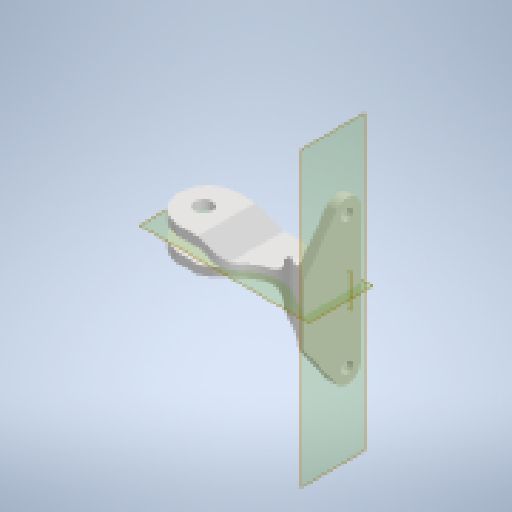
# Autodesk Inventor part: AcopleCamara-part2
Saved by Autodesk Inventor 2023 (Build 270158000, 158)
## iProperties
Created: 2023-12-18
Part Number: AcopleCamara-part2
Material: Genérico
Document SubType Name: Modeling
Designer: ASUS
Density: 1 g/cm^3
Appearance: Valor por defecto
Author: ASUS
Autodesk Inventor part; units mm, degrees
ref_plane "YZ Plane" through (0, 0, 0) normal (1, 0, 0) x (0, 1, 0)
ref_plane "XZ Plane" through (0, 0, 0) normal (0, 1, 0) x (-1, 0, 0)
ref_plane "XY Plane" through (0, 0, 0) normal (0, 0, 1) x (1, 0, 0)
ref_plane "Plano de trabajo1" through (-5.5, 31.0579, -5.3088) normal (0, 0, -1) x (0, -1, 0)
sketch "Boceto1" plane through (0, 0, -5.3088) normal (0, 0, 1) x (1, 0, 0)
  line L0 (-3, 28.0579) -> (-10.9599, 26.1093) projected
  line L1 (-3, 34.0579) -> (-3, 28.0579) projected
  line L2 (-10.9599, 36.0066) -> (-3, 34.0579) projected
  line L3 (-10.9599, 26.1093) -> (-10.9599, 36.0066) projected
  line L4 (-3, 34.0579) -> (-3, 62.1159) projected
  line L5 (-3, 0) -> (-3, 28.0579) projected
  line L6 (-11.1599, 36.2645) -> (-11.1599, 25.8544)
  line L7 (-3.2, 0) -> (-3.2, 28.009)
  line L8 (-3.2, 28.009) -> (-3.2, 28.0579)
  line L9 (-11.1599, 25.8544) -> (-3.2, 27.8031)
  line L10 (-3, 27.852) -> (-2.9524, 27.8637)
  line L11 (-3.2, 34.0579) -> (-3.2, 34.1069)
  line L12 (-3.2, 28.0579) -> (-3.2, 62.1189)
  line L13 (-2.9524, 34.2522) -> (-3, 34.2638)
  line L14 (-3.2, 34.3159) -> (-11.1599, 36.2645)
  arc A0 (-60.3157, 26.6827) -> (-60.3209, 35.4723) centre (-90.5, 31.0595) ccw projected
  arc A1 (-57.3658, 26.1226) -> (-57.3864, 36.1324) centre (-90.5, 31.0595) ccw projected
  line L15 (-60, 31.0595) -> (-57, 31.0595) construction
  line L16 (-12.8167, 21.8544) -> (-3.2, 21.8544)
  line L17 (-15.1599, 24.1976) -> (-15.1599, 37.9214)
  line L18 (-12.8167, 21.8544) -> (-15.1599, 24.1976)
  line L19 (-12.8167, 40.2645) -> (-3.2, 40.2645)
  line L20 (-12.8167, 40.2645) -> (-15.1599, 37.9214)
  line L21 (-57, 31.0595) -> (-11.1599, 31.0595) construction
  line L22 (-52.0001, 29.0595) -> (-52.0001, 33.0595)
  line L23 (-52.0001, 28.7595) -> (-37.0001, 28.7595)
  line L24 (-47.0001, 29.0595) -> (-42.0001, 29.0595)
  line L25 (-42.0001, 29.0595) -> (-42.0001, 33.0595)
  line L26 (-42.0001, 33.0595) -> (-47.0001, 33.0595)
  line L27 (-47.0001, 33.0595) -> (-47.0001, 29.0595)
  line L28 (-52.0001, 25.7595) -> (-37.0001, 25.7595)
  line L29 (-52.0001, 25.7595) -> (-52.0001, 28.7595)
  line L30 (-37.0001, 28.7595) -> (-37.0001, 33.0595) construction
  line L31 (-37.0001, 28.7595) -> (-36.5001, 28.7595)
  line L32 (-37.0001, 25.7595) -> (-27.9334, 29.0595)
  line L33 (-52.0001, 29.0595) -> (-37.0001, 29.0595)
  line L34 (-27.9334, 29.0595) -> (-15.1599, 29.0595)
  line L35 (-52.0001, 33.3595) -> (-37.0001, 33.3595)
  line L36 (-52.0001, 36.3595) -> (-37.0001, 36.3595)
  line L37 (-52.0001, 36.3595) -> (-52.0001, 33.3595)
  line L38 (-37.0001, 33.3595) -> (-36.5001, 33.3595)
  line L39 (-37.0001, 36.3595) -> (-27.9334, 33.0595)
  line L40 (-52.0001, 33.0595) -> (-37.0001, 33.0595)
  line L41 (-27.9334, 33.0595) -> (-15.1599, 33.0595)
  line L42 (-36.5001, 28.7595) -> (-30.1809, 31.0595)
  line L43 (-36.5001, 33.3595) -> (-30.1809, 31.0595)
  point P0 (0, 0)
  point P1 (-57.0001, 31.1283)
  point P2 (-47.0001, 31.0595)
  dimension "d0" = 0.2
  dimension "d3" = 4
  dimension "d7" = 4
  dimension "d9" = 4
  dimension "d10" = 5
  dimension "d12" = 5
  dimension "d13" = 5
  dimension "d14" = 15
  dimension "d15" = 3
  constraints: 76 end point, 16 parallel, 14 point on line, 10 symmetric about line, 9 horizontal, 5 vertical, 3 point on circle, 2 midpoint, 2 perpendicular, 1 other
  measures "d0" distance between parallel lines of L3 L6
  measures "d3" distance from line of L6.end L16
  measures "d7" distance between parallel lines of L6 L17
  measures "d9" distance from line of L6.end L18
  measures "d10" distance from line of point (-57, 31.128) L22
  measures "d12" distance of L26.end L25.end
  measures "d13" distance between parallel lines of L22 L27
  measures "d14" distance of L23.start L23.end
  measures "d15" distance between parallel lines of L23 L28
extrude "Extrusión1" add sketch "Boceto1" against normal blind 4 contours L7 L9 L6 L14 L12 L2 L3 L0 | L0 L3 L2 L11 L12 L8 | L7 L16 L18 L17 L20 L19 L12 L14 L6 L9 | L34 L32 L28 L29 L23 L31 L42 L43 L38 L35 L37 L36 L39 L41 L17
extrude "Extrusión2" add sketch "Boceto1" along normal blind 14.5 contours L7 L16 L18 L17 L20 L19 L12 L14 L6 L9 | L34 L32 L28 L29 L23 L31 L42 L43 L38 L35 L37 L36 L39 L41 L17
ref_plane "Plano de trabajo2" through (-3, 31.0579, 0) normal (-1, 0, 0) x (0, 0, 1)
sketch "Boceto2" plane through (-3.2, 31.0579, 0) normal (-1, 0, 0) x (0, 0, 1)
  circle A0 centre (-4.8054, -21.2007) radius 1.75
  circle A1 centre (-4.7908, 21.2015) radius 1.75
  line L0 (-9.3092, -9.2035) -> (9.1912, -9.2035)
  arc A2 (-9.3092, -21.2007) -> (-1.1279, -23.8005) centre (-4.8054, -21.2007) ccw
  line L1 (-1.1279, -23.8005) -> (9.1912, -9.2035)
  arc A3 (-1.1279, -23.8005) -> (-9.3092, -21.2007) centre (-4.8054, -21.2007) ccw construction
  line L2 (-9.3088, 3) -> (-9.3088, -3)
  line L3 (-9.3088, 0) -> (9.1912, 0.0015) construction
  line L4 (9.1912, -5.2035) -> (9.1912, 5.2066)
  line L5 (-9.3092, 9.2035) -> (-9.3092, -21.2007)
  line L6 (-9.3107, 9.2035) -> (9.1896, 9.2066)
  arc A4 (-1.1318, 23.8018) -> (-9.3127, 21.2007) centre (-4.809, 21.2014) ccw
  line L7 (-1.1318, 23.8018) -> (9.1896, 9.2066)
  line L8 (-9.3107, 9.2035) -> (-9.3127, 21.2007)
  point P0 (-9.3088, -9.2035)
  point P1 (-9.3104, 9.2035)
  constraints: 18 end point, 8 point on line, 6 point on circle, 5 centre point, 2 midpoint
extrude "Extrusión3" add sketch "Boceto2" along normal blind 3 contours A0 | A1 | L0 L1 A2 L5 | L8 A4 L7 L6
sketch "Boceto3" plane through (-6.2, 31.0579, 0) normal (-1, 0, 0) x (0, 0, 1)
  circle A0 centre (-4.8054, -21.2007) radius 1.75 projected
  circle A1 centre (-4.7908, 21.2015) radius 1.75 projected
  point P0 (0, -31.0579)
hole "Agujero1" at (-6.2, 9.8572, -4.8054) at (-6.2, 52.2595, -4.7908) direction (1, 0, 0) diameter 3.5 end through all countersink diameter 6 countersink angle 90
fillet "Empalme1" radius 5 4 edges at (-6.2, 21.8544, -0.0588) (-6.2, 40.2645, -0.0596) (-15.1599, 33.0595, -0.0588) (-15.1599, 29.0595, -0.0588)
ref_plane "Plano de trabajo3" through (-52.0001, 31.0595, -9.3088) normal (0, -1, 0) x (1, 0, 0)
sketch "Boceto4" plane through (-52.0001, 31.0595, -9.3088) normal (0, -1, 0) x (1, 0, 0)
  line L0 (0, 0) -> (0, 18.5)
  line L1 (0, 18.5) -> (15.5, 18.5)
  line L2 (48.8001, 8.181) -> (48.8001, -0.0004)
  line L3 (48.8001, -0.0004) -> (45.8001, -0.0004)
  line L4 (48.8001, 4) -> (48.8001, 0)
  line L5 (48.8001, 0) -> (0, 0)
  line L6 (0, 0) -> (0, 18.5)
  line L7 (0, 18.5) -> (48.8001, 18.5)
  line L8 (48.8001, 18.5) -> (48.8001, 0)
  line L9 (49.0001, 18.618) -> (40.8402, 13.9069)
  line L10 (24.0667, 0) -> (24.0667, 18.5)
  line L11 (40.8402, 4) -> (40.8402, 18.5)
  arc A0 (24.0667, 18.5) -> (40.8402, 13.9069) centre (34.725, 24.4988) ccw
  point P0 (52.0001, 9.3088)
  point P1 (48.7957, 18.5)
  constraints: 24 end point, 2 point on circle, 1 centre point, 1 point on line
extrude "Extrusión4" cut sketch "Boceto4" along normal through all both and the other way through all contours L7 L11 A0 | L7 L9 L11
fillet "Empalme2" radius 10 1 edges at (-27.9334, 31.0595, 9.1912)
sketch "Boceto5" plane through (-52.0001, 31.0595, -9.3088) normal (0, -1, 0) x (1, 0, 0)
  line L0 (0, 0) -> (0, 18.5) projected
  line L1 (15.5, 0) -> (0, 0) projected
  line L2 (15.5, 0) -> (15.5, 18.5) projected
  line L3 (0, 18.5) -> (15.5, 18.5) projected
  line L4 (0, 0) -> (15, 0) projected
  line L5 (0, 0) -> (15.5, 18.5) construction
  line L6 (0, 18.5) -> (15.5, 0) construction
  circle A0 centre (7.75, 9.25) radius 2.75
  point P0 (52.0001, 9.3088)
  dimension "d42" = 5.5
  constraints: 4 end point, 1 centre point, 1 midpoint
  measures "d42" diameter of A0
extrude "Extrusión5" cut sketch "Boceto5" along normal through all both and the other way through all contours A0
fillet "Empalme3" radius 9 4 edges at (-52.0001, 27.2595, 9.1912) (-52.0001, 27.2595, -9.3088) (-52.0001, 34.8595, -9.3088) (-52.0001, 34.8595, 9.1912)
fillet "Empalme4" radius 0.5 1 edges at (-30.1809, 31.0595, -0.2214)
